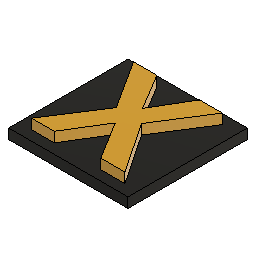
icon_active (Autodesk Fusion 360 design; units mm, degrees)
Autodesk Fusion 360 part; units mm, degrees
sketch "Sketch1" plane through (0, 0, 0) normal (0, 0, 1) x (1, 0, 0)
  line L0 (5.95, -5.95) -> (-5.95, -5.95)
  line L1 (-5.95, -5.95) -> (-5.95, 5.95)
  line L2 (-5.95, 5.95) -> (5.95, 5.95)
  line L3 (5.95, 5.95) -> (5.95, -5.95)
  line L4 (5.95, -5.95) -> (-5.95, 5.95) construction
  line L5 (-5.95, -5.95) -> (5.95, 5.95) construction
  line L6 (4.6526, -4.9591) -> (2.2411, -4.9591)
  line L7 (2.2411, -4.9591) -> (-0.0749, -1.1921)
  line L8 (-0.0749, -1.1921) -> (-2.391, -4.9591)
  line L9 (-2.391, -4.9591) -> (-4.6526, -4.9591)
  line L10 (-4.6526, -4.9591) -> (-1.3488, 0.1771)
  line L11 (-1.3488, 0.1771) -> (-4.4414, 5)
  line L12 (-4.4414, 5) -> (-2.1117, 5)
  line L13 (-2.1117, 5) -> (0.0341, 1.4169)
  line L14 (0.0341, 1.4169) -> (2.139, 5)
  line L15 (2.139, 5) -> (4.4142, 5)
  line L16 (4.4142, 5) -> (1.2875, 0.0613)
  line L17 (1.2875, 0.0613) -> (4.6526, -4.9591)
  dimension "d1" = 11.9
  dimension "d2" = 11.9
  constraint perpendicular L0 L1
  measures "d1" distance of L1.end L2.end
  measures "d2" distance of L0.end L1.end
extrude "Extrude1" add sketch "Sketch1" against normal blind 1 contours L0 L1 L2 L3 | L6 L7 L8 L9 L10 L11 L12 L13 L14 L15 L16 L17
extrude "Extrude3" add sketch "Sketch1" along normal blind 1 contours L6 L7 L8 L9 L10 L11 L12 L13 L14 L15 L16 L17
